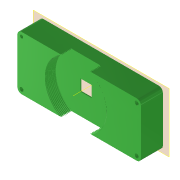
# Autodesk Inventor part: OutputFile
Saved by Autodesk Inventor 2022 (Build 260153000, 153)
## iProperties
Created: 2022-02-02
Part Number: OutputFile
Material: Generisch
Document SubType Name: Modeling
Designer: diederichbenedict
Density: 1 g/cm^3
Appearance: Glatt - Waldgrün
Mass: 24.3371 g
Surface Area: 140.293 cm^2
Volume: 24.3371 cm^3
Author: diederichbenedict
Autodesk Inventor part; units mm, degrees
ref_plane "YZ Plane" through (0, 0, 0) normal (1, 0, 0) x (0, 1, 0)
ref_plane "XZ Plane" through (0, 0, 0) normal (0, 1, 0) x (-1, 0, 0)
ref_plane "XY Plane" through (0, 0, 0) normal (0, 0, 1) x (1, 0, 0)
ref_plane "Arbeitsebene1" through (0, 0, 0) normal (0, 0, 1) x (1, 0, 0)
sketch "Skizze1" plane through (0, 0, 0) normal (0, 0, 1) x (1, 0, 0)
  line L0 (55.3299, 14.4874) -> (55.3299, -14.4874)
  line L1 (55.3299, -14.4874) -> (-23.745, -14.4874)
  line L2 (-23.745, -14.4874) -> (-23.745, 14.4874)
  line L3 (-23.745, 14.4874) -> (55.3299, 14.4874)
  line L4 (-3.798, -8.3739) -> (-3.798, -13.5126) projected
  line L5 (26.202, -8.3739) -> (-3.798, -8.3739) projected
  line L6 (-3.865, 8.7531) -> (26.135, 8.7531) projected
  line L7 (-3.865, 13.4874) -> (-3.865, 8.7531) projected
  line L8 (-3.865, 13.4874) -> (-14.255, 13.4874) projected
  arc A0 (-14.255, 13.4874) -> (-15.255, 12.4874) centre (-14.255, 12.4874) ccw projected
  line L9 (-15.255, 12.4874) -> (-15.255, -12.5126) projected
  arc A1 (-15.255, -12.5126) -> (-14.255, -13.5126) centre (-14.255, -12.5126) ccw projected
  line L10 (-14.255, -13.5126) -> (-3.798, -13.5126) projected
  arc A2 (-18.955, -12.5126) -> (-14.255, -17.2126) centre (-14.255, -12.5126) ccw projected
  line L11 (-18.955, -12.5126) -> (-18.955, 12.4874) projected
  arc A3 (-14.255, 17.1874) -> (-18.955, 12.4874) centre (-14.255, 12.4874) ccw projected
  line L12 (-14.255, 17.1874) -> (23.745, 17.1874) projected
  arc A4 (28.445, 12.4874) -> (23.745, 17.1874) centre (23.745, 12.4874) ccw projected
  arc A5 (23.745, -17.2126) -> (28.445, -12.5126) centre (23.745, -12.5126) ccw projected
  line L13 (23.745, -17.2126) -> (-14.255, -17.2126) projected
  circle A6 centre (57.3299, 16.4874) radius 1.4 projected
  circle A7 centre (-25.745, -16.4874) radius 1.4 projected
  circle A8 centre (57.3299, -16.4874) radius 1.4 projected
  circle A9 centre (-25.745, 16.4874) radius 1.15 projected
  line L14 (60.3299, 16.4874) -> (60.3299, -16.4874) projected
  arc A10 (60.3299, 16.4874) -> (57.3299, 19.4874) centre (57.3299, 16.4874) ccw projected
  line L15 (-25.745, 19.4874) -> (57.3299, 19.4874) projected
  arc A11 (-25.745, 19.4874) -> (-28.745, 16.4874) centre (-25.745, 16.4874) ccw projected
  line L16 (-28.745, -16.4874) -> (-28.745, 16.4874) projected
  arc A12 (-28.745, -16.4874) -> (-25.745, -19.4874) centre (-25.745, -16.4874) ccw projected
  line L17 (57.3299, -19.4874) -> (-25.745, -19.4874) projected
  arc A13 (57.3299, -19.4874) -> (60.3299, -16.4874) centre (57.3299, -16.4874) ccw projected
  arc A14 (-18.955, -12.5126) -> (-14.255, -17.2126) centre (-14.255, -12.5126) ccw projected
  line L18 (-18.955, -12.5126) -> (-18.955, 12.4874) projected
  arc A15 (-14.255, 17.1874) -> (-18.955, 12.4874) centre (-14.255, 12.4874) ccw projected
  line L19 (-14.255, 17.1874) -> (23.745, 17.1874) projected
  arc A16 (28.445, 12.4874) -> (23.745, 17.1874) centre (23.745, 12.4874) ccw projected
  line L20 (28.445, 12.4874) -> (26.135, 12.4874) projected
  line L21 (26.135, 8.7531) -> (26.135, 12.4874) projected
  line L22 (26.202, -12.5126) -> (26.202, -8.3739) projected
  line L23 (26.202, -12.5126) -> (28.445, -12.5126) projected
  arc A17 (23.745, -17.2126) -> (28.445, -12.5126) centre (23.745, -12.5126) ccw projected
  line L24 (23.745, -17.2126) -> (-14.255, -17.2126) projected
  circle A18 centre (57.3299, 16.4874) radius 1.4 projected
  circle A19 centre (-25.745, -16.4874) radius 1.4 projected
  circle A20 centre (57.3299, -16.4874) radius 1.4 projected
  circle A21 centre (-25.745, 16.4874) radius 1.15 projected
  line L25 (60.3299, 16.4874) -> (60.3299, -16.4874) projected
  arc A22 (60.3299, 16.4874) -> (57.3299, 19.4874) centre (57.3299, 16.4874) ccw projected
  line L26 (-25.745, 19.4874) -> (57.3299, 19.4874) projected
  arc A23 (-25.745, 19.4874) -> (-28.745, 16.4874) centre (-25.745, 16.4874) ccw projected
  line L27 (-28.745, -16.4874) -> (-28.745, 16.4874) projected
  arc A24 (-28.745, -16.4874) -> (-25.745, -19.4874) centre (-25.745, -16.4874) ccw projected
  line L28 (57.3299, -19.4874) -> (-25.745, -19.4874) projected
  arc A25 (57.3299, -19.4874) -> (60.3299, -16.4874) centre (57.3299, -16.4874) ccw projected
  line L29 (28.445, 12.4874) -> (26.135, 12.4874) projected
  line L30 (26.135, 8.7531) -> (26.135, 12.4874) projected
  line L31 (-3.865, 8.7531) -> (26.135, 8.7531) projected
  line L32 (-3.865, 13.4874) -> (-3.865, 8.7531) projected
  line L33 (-3.865, 13.4874) -> (-14.255, 13.4874) projected
  arc A26 (-14.255, 13.4874) -> (-15.255, 12.4874) centre (-14.255, 12.4874) ccw projected
  line L34 (-15.255, 12.4874) -> (-15.255, -12.5126) projected
  arc A27 (-15.255, -12.5126) -> (-14.255, -13.5126) centre (-14.255, -12.5126) ccw projected
  line L35 (-14.255, -13.5126) -> (-3.798, -13.5126) projected
  line L36 (-3.798, -8.3739) -> (-3.798, -13.5126) projected
  line L37 (26.202, -8.3739) -> (-3.798, -8.3739) projected
  line L38 (26.202, -12.5126) -> (26.202, -8.3739) projected
  line L39 (26.202, -12.5126) -> (28.445, -12.5126) projected
  point P0 (0, 0)
  point P1 (-15.255, 11.1874)
  point P2 (28.01, -14.4874)
  point P3 (-18.5199, -14.4874)
  point P4 (-18.5082, 14.4874)
  point P5 (27.9983, 14.4874)
  constraints: 8 end point
ref_plane "Arbeitsebene2" through (-3.9015, -6.25, 7.6898) normal (0, 0, 1) x (1, 0, 0)
extrude "Extrusion1" add sketch "Skizze1" along normal up to surface (7.6898 mm away)
sketch "Skizze2" plane through (-25.745, -19.4874, 7.6898) normal (0, 0, 1) x (1, 0, 0)
  line L0 (34.9935, 15.3874) -> (43.1935, 15.3874)
  line L1 (43.1935, 15.3874) -> (43.1935, 23.5874)
  line L2 (43.1935, 23.5874) -> (34.9935, 23.5874)
  line L3 (34.9935, 23.5874) -> (34.9935, 15.3874)
  line L4 (34.9935, 15.3874) -> (43.1935, 23.5874) construction
  line L5 (43.1935, 15.3874) -> (34.9935, 23.5874) construction
  line L6 (81.0749, 33.9749) -> (53.7433, 33.9749) projected
  line L7 (81.0749, 5) -> (81.0749, 33.9749) projected
  line L8 (53.755, 5) -> (81.0749, 5) projected
  arc A0 (49.4901, 2.2749) -> (53.755, 5) centre (49.4901, 6.9749) ccw projected
  line L9 (11.4901, 2.2749) -> (49.4901, 2.2749) projected
  arc A1 (7.2251, 5) -> (11.4901, 2.2749) centre (11.4901, 6.9749) ccw projected
  line L10 (2, 5) -> (7.2251, 5) projected
  line L11 (2, 33.9749) -> (2, 5) projected
  line L12 (7.2369, 33.9749) -> (2, 33.9749) projected
  arc A2 (11.4901, 36.6749) -> (7.2369, 33.9749) centre (11.4901, 31.9749) ccw projected
  line L13 (49.4901, 36.6749) -> (11.4901, 36.6749) projected
  arc A3 (53.7433, 33.9749) -> (49.4901, 36.6749) centre (49.4901, 31.9749) ccw projected
  circle A4 centre (83.0749, 35.9749) radius 1.4 projected
  circle A5 centre (0, 3) radius 1.4 projected
  circle A6 centre (83.0749, 3) radius 1.4 projected
  circle A7 centre (0, 35.9749) radius 1.15 projected
  arc A8 (0, 38.9749) -> (-3, 35.9749) centre (0, 35.9749) ccw projected
  line L14 (-3, 3) -> (-3, 35.9749) projected
  arc A9 (-3, 3) -> (0, 0) centre (0, 3) ccw projected
  line L15 (83.0749, 0) -> (0, 0) projected
  arc A10 (83.0749, 0) -> (86.0749, 3) centre (83.0749, 3) ccw projected
  line L16 (86.0749, 35.9749) -> (86.0749, 3) projected
  arc A11 (86.0749, 35.9749) -> (83.0749, 38.9749) centre (83.0749, 35.9749) ccw projected
  line L17 (0, 38.9749) -> (83.0749, 38.9749) projected
  circle A12 centre (39.0935, 19.4874) radius 3.6158 projected
  point P0 (25.745, 19.4874)
  dimension "d3" = 8.2
  dimension "d4" = 8.2
  constraints: 12 end point, 2 parallel, 1 horizontal, 1 perpendicular
  measures "d3" distance of L2.end L1.end
  measures "d4" distance of L1.end L0.end
extrude "Extrusion2" add sketch "Skizze2" along normal blind 2.2 contours L7 L8 A0 L9 A1 L10 L11 L12 A2 L13 A3 L6 | L17 A11 L16 A10 L15 A9 L14 A8
ref_plane "Arbeitsebene3" through (-21.9576, -12.7, 16.9028) normal (0, 0, -1) x (0, 1, 0)
sketch "Skizze3" plane through (-25.745, -19.4874, 9.8898) normal (0, 0, 1) x (1, 0, 0)
  line L0 (34.9935, 15.3874) -> (34.9935, 23.5874) projected
  line L1 (34.9935, 23.5874) -> (43.1935, 23.5874) projected
  line L2 (43.1935, 23.5874) -> (43.1935, 15.3874) projected
  line L3 (43.1935, 15.3874) -> (34.9935, 15.3874) projected
  circle A0 centre (39.0935, 19.4874) radius 3.6158 projected
  circle A1 centre (39.0935, 19.4874) radius 3.475
  line L4 (83.0749, 38.9749) -> (0, 38.9749) projected
  arc A2 (0, 38.9749) -> (-3, 35.9749) centre (0, 35.9749) ccw projected
  line L5 (-3, 35.9749) -> (-3, 3) projected
  arc A3 (-3, 3) -> (0, 0) centre (0, 3) ccw projected
  line L6 (0, 0) -> (83.0749, 0) projected
  arc A4 (83.0749, 0) -> (86.0749, 3) centre (83.0749, 3) ccw projected
  line L7 (86.0749, 3) -> (86.0749, 35.9749) projected
  arc A5 (86.0749, 35.9749) -> (83.0749, 38.9749) centre (83.0749, 35.9749) ccw projected
  line L8 (34.9935, 15.3874) -> (34.9935, 23.5874) projected
  line L9 (34.9935, 23.5874) -> (43.1935, 23.5874) projected
  line L10 (43.1935, 23.5874) -> (43.1935, 15.3874) projected
  line L11 (43.1935, 15.3874) -> (34.9935, 15.3874) projected
  circle A6 centre (0, 35.9749) radius 1.15 projected
  circle A7 centre (83.0749, 3) radius 1.4 projected
  circle A8 centre (0, 3) radius 1.4 projected
  circle A9 centre (83.0749, 35.9749) radius 1.4 projected
  point P0 (25.745, 19.4874)
  dimension "d7" = 6.95
  constraints: 1 centre point, 1 coincident
  measures "d7" diameter of A1
extrude "Extrusion3" add sketch "Skizze3" along normal blind 6 contours L0 L1 L2 L3 | A5 L7 A4 L6 A3 L5 A2 L4
sketch "Skizze4" plane through (-25.745, 19.4874, 15.8898) normal (0, 0, 1) x (1, 0, 0)
  circle A0 centre (39.0935, -19.4874) radius 3.6158 projected
  circle A1 centre (39.0935, -19.4874) radius 22
  point P0 (25.745, -19.4874)
  dimension "d10" = 44
  constraints: 1 centre point, 1 coincident
  measures "d10" diameter of A1
extrude "Extrusion4" cut sketch "Skizze4" against normal blind 7.5
sketch "Sketch7" plane through (13.3485, 22.5, 5.8898) normal (-1, 0, 0) x (0, 0, 1)
  line L0 (2.5, 0.2165) -> (2.3389, -0.0625) construction
  line L1 (2.5, 0.2165) -> (2.6611, -0.0625) construction
  line L2 (2.5, 0.2165) -> (2.5, 0) construction
  line L3 (2.375, 0) -> (2.4472, 0) construction
  line L4 (3, -0.6495) -> (3.0625, -0.5413) construction
  line L5 (2, -0.6495) -> (1.9375, -0.5413) construction
  line L6 (1.9375, -0.5413) -> (2, -0.5413) construction
  line L7 (2.0625, -0.5413) -> (2, -0.6495) construction
  arc A0 (2.4472, 0) -> (2.3389, -0.0625) centre (2.4472, -0.125) ccw
  arc A1 (2.6611, -0.0625) -> (2.5528, 0) centre (2.5528, -0.125) ccw
  line L8 (3, -0.6495) -> (3, -0.5413) construction
  line L9 (2, -0.6495) -> (2, -0.5413) construction
  arc A2 (2.9195, -0.51) -> (2.9736, -0.5413) centre (2.9736, -0.4788) ccw
  line L10 (2.6611, -0.0625) -> (2.9195, -0.51)
  line L11 (2.4472, 0) -> (2.5528, 0)
  line L12 (2.3389, -0.0625) -> (2.0805, -0.51)
  line L13 (2.9736, -0.5413) -> (3, -0.5413) construction
  line L14 (3, -0.5413) -> (3.0625, -0.5413) construction
  arc A3 (2.0264, -0.5413) -> (2.0805, -0.51) centre (2.0264, -0.4788) ccw
  line L15 (2.0805, -0.51) -> (2.0625, -0.5413) construction
  line L16 (2, -0.5413) -> (2.0264, -0.5413) construction
  line L17 (2.0264, -0.5413) -> (2.9736, -0.5413)
  line L18 (0, 0) -> (0.4413, 0)
  line L19 (0, 0) -> (0, 0.419)
  line L20 (3, -0.6495) -> (2.9195, -0.51) construction
  dimension "d41" = 0.2165
  dimension "d42" = 0.125
  dimension "d43" = 0.0625
  dimension "d44" = 0.1082
  dimension "d45" = 1
  dimension "Sketch7_MajorRadius" = 0.5413
  dimension "d47" = 60
  dimension "Sketch7_ThreadOffset" = 3
  dimension "Sketch7_MinorRadius" = 0
  constraints: 42 end point, 17 tangent, 8 point on circle, 6 parallel, 5 collinear, 4 centre point, 3 point on line, 2 equal radius, 2 horizontal, 2 perpendicular, 2 vertical, 1 equal length, 1 midpoint, 4 other
  measures "d41" distance from line of L0.start L3
  measures "d42" radius of A0
  measures "d43" radius of A2
  measures "d44" distance from line of L14 L4.start
  measures "d45" distance between parallel lines of L8 L9
  measures "Sketch7_MajorRadius" distance between parallel lines of L14 L18
  measures "d47" angle of L10 L12
  measures "Sketch7_ThreadOffset" distance between parallel lines of L19 L8
  measures "Sketch7_MinorRadius" distance between parallel lines of L18 L11
thread "Gewinde1" size "M45x1" class "6H" standard "ANSI Metric M Profile" full length
sketch "Skizze10" plane through (-25.745, -19.4874, 7.6898) normal (0, 0, -1) x (-1, 0, 0)
  arc A0 (-50.4901, 6.9749) -> (-49.4901, 5.9749) centre (-49.4901, 6.9749) ccw projected
  line L0 (-49.4901, 5.9749) -> (-11.4901, 5.9749) projected
  arc A1 (-11.4901, 5.9749) -> (-10.4901, 6.9749) centre (-11.4901, 6.9749) ccw projected
  line L1 (-10.4901, 6.9749) -> (-10.4901, 31.9749) projected
  arc A2 (-10.4901, 31.9749) -> (-11.4901, 32.9749) centre (-11.4901, 31.9749) ccw projected
  line L2 (-11.4901, 32.9749) -> (-49.4901, 32.9749) projected
  arc A3 (-49.4901, 32.9749) -> (-50.4901, 31.9749) centre (-49.4901, 31.9749) ccw projected
  line L3 (-50.4901, 31.9749) -> (-50.4901, 6.9749) projected
  line L4 (3, 35.9749) -> (3, 3) projected
  arc A4 (3, 35.9749) -> (0, 38.9749) centre (0, 35.9749) ccw projected
  line L5 (-83.0749, 38.9749) -> (0, 38.9749) projected
  arc A5 (-83.0749, 38.9749) -> (-86.0749, 35.9749) centre (-83.0749, 35.9749) ccw projected
  line L6 (-86.0749, 3) -> (-86.0749, 35.9749) projected
  arc A6 (-86.0749, 3) -> (-83.0749, 0) centre (-83.0749, 3) ccw projected
  line L7 (0, 0) -> (-83.0749, 0) projected
  arc A7 (0, 0) -> (3, 3) centre (0, 3) ccw projected
  circle A8 centre (0, 35.9749) radius 1.15 projected
  circle A9 centre (-83.0749, 3) radius 1.4 projected
  circle A10 centre (0, 3) radius 1.4 projected
  circle A11 centre (-83.0749, 35.9749) radius 1.4 projected
  line L8 (-81.0749, 33.9749) -> (-81.0749, 5) projected
  line L9 (-53.7433, 33.9749) -> (-81.0749, 33.9749) projected
  arc A12 (-49.4901, 36.6749) -> (-53.7433, 33.9749) centre (-49.4901, 31.9749) ccw projected
  line L10 (-11.4901, 36.6749) -> (-49.4901, 36.6749) projected
  arc A13 (-7.2369, 33.9749) -> (-11.4901, 36.6749) centre (-11.4901, 31.9749) ccw projected
  line L11 (-2, 33.9749) -> (-7.2369, 33.9749) projected
  line L12 (-2, 5) -> (-2, 33.9749) projected
  line L13 (-7.2251, 5) -> (-2, 5) projected
  arc A14 (-11.4901, 2.2749) -> (-7.2251, 5) centre (-11.4901, 6.9749) ccw projected
  line L14 (-49.4901, 2.2749) -> (-11.4901, 2.2749) projected
  arc A15 (-53.755, 5) -> (-49.4901, 2.2749) centre (-49.4901, 6.9749) ccw projected
  line L15 (-81.0749, 5) -> (-53.755, 5) projected
  line L16 (-6.7901, 31.9749) -> (-6.7901, 6.9749)
  arc A16 (-11.4901, 2.2749) -> (-6.7901, 6.9749) centre (-11.4901, 6.9749) ccw
  line L17 (-11.4901, 2.2749) -> (-49.4901, 2.2749)
  arc A17 (-54.1901, 6.9749) -> (-49.4901, 2.2749) centre (-49.4901, 6.9749) ccw
  line L18 (-54.1901, 6.9749) -> (-54.1901, 31.9749)
  arc A18 (-49.4901, 36.6749) -> (-54.1901, 31.9749) centre (-49.4901, 31.9749) ccw
  line L19 (-49.4901, 36.6749) -> (-11.4901, 36.6749)
  arc A19 (-6.7901, 31.9749) -> (-11.4901, 36.6749) centre (-11.4901, 31.9749) ccw
  line L20 (-10.6401, 31.9749) -> (-10.6401, 6.9749)
  arc A20 (-11.4901, 6.1249) -> (-10.6401, 6.9749) centre (-11.4901, 6.9749) ccw
  line L21 (-11.4901, 6.1249) -> (-49.4901, 6.1249)
  arc A21 (-50.3401, 6.9749) -> (-49.4901, 6.1249) centre (-49.4901, 6.9749) ccw
  line L22 (-50.3401, 6.9749) -> (-50.3401, 31.9749)
  arc A22 (-49.4901, 32.8249) -> (-50.3401, 31.9749) centre (-49.4901, 31.9749) ccw
  line L23 (-49.4901, 32.8249) -> (-11.4901, 32.8249)
  arc A23 (-10.6401, 31.9749) -> (-11.4901, 32.8249) centre (-11.4901, 31.9749) ccw
  point P0 (-25.745, 19.4874)
  point P1 (-53.755, 5)
  dimension "d72" = 0.15
  constraints: 17 point on circle, 16 end point, 8 centre point, 14 other
  measures "d72" distance between parallel lines of L1 L20
extrude "Extrusion6" add sketch "Skizze10" along normal blind 3 contours L3 A3 L2 A2 L1 A1 L0 A0 | A12 L10 A13 A19 L16 A16 A14 L14 A15 A17 L18 A18
coil "Spirale4" sketch "Sketch7" operation cut axis through (13.3485, 0, 15.8898) along (0, 0, 1) pitch 1.001 turns 9.99001 hand right
sketch "Skizze11" plane through (-25.745, -19.4874, 4.6898) normal (0, 0, -1) x (-1, 0, 0)
  arc A0 (-6.7901, 31.9749) -> (-7.2369, 33.9749) centre (-11.4901, 31.9749) ccw projected
  arc A1 (-7.2369, 33.9749) -> (-11.4901, 36.6749) centre (-11.4901, 31.9749) ccw projected
  line L0 (-49.4901, 36.6749) -> (-11.4901, 36.6749) projected
  arc A2 (-49.4901, 36.6749) -> (-53.7433, 33.9749) centre (-49.4901, 31.9749) ccw projected
  arc A3 (-53.7433, 33.9749) -> (-54.1901, 31.9749) centre (-49.4901, 31.9749) ccw projected
  line L1 (-54.1901, 31.9749) -> (-54.1901, 6.9749) projected
  arc A4 (-54.1901, 6.9749) -> (-53.755, 5) centre (-49.4901, 6.9749) ccw projected
  arc A5 (-53.755, 5) -> (-49.4901, 2.2749) centre (-49.4901, 6.9749) ccw projected
  line L2 (-11.4901, 2.2749) -> (-49.4901, 2.2749) projected
  arc A6 (-11.4901, 2.2749) -> (-7.2251, 5) centre (-11.4901, 6.9749) ccw projected
  arc A7 (-7.2251, 5) -> (-6.7901, 6.9749) centre (-11.4901, 6.9749) ccw projected
  line L3 (-6.7901, 6.9749) -> (-6.7901, 31.9749) projected
  line L4 (-49.4901, 32.8249) -> (-11.4901, 32.8249) projected
  arc A8 (-10.6401, 31.9749) -> (-11.4901, 32.8249) centre (-11.4901, 31.9749) ccw projected
  line L5 (-10.6401, 31.9749) -> (-10.6401, 6.9749) projected
  arc A9 (-11.4901, 6.1249) -> (-10.6401, 6.9749) centre (-11.4901, 6.9749) ccw projected
  line L6 (-11.4901, 6.1249) -> (-49.4901, 6.1249) projected
  arc A10 (-50.3401, 6.9749) -> (-49.4901, 6.1249) centre (-49.4901, 6.9749) ccw projected
  line L7 (-50.3401, 6.9749) -> (-50.3401, 31.9749) projected
  arc A11 (-49.4901, 32.8249) -> (-50.3401, 31.9749) centre (-49.4901, 31.9749) ccw projected
  line L8 (-54.1901, 31.9749) -> (-54.1901, 6.9749) projected
  line L9 (-54.1901, 31.9749) -> (-50.3401, 31.9749)
  line L10 (-50.3401, 31.9749) -> (-50.3401, 6.9749)
  line L11 (-50.3401, 6.9749) -> (-54.1901, 6.9749)
  line L12 (-54.1901, 6.9749) -> (-54.1901, 31.9749)
  point P0 (-25.745, 19.4874)
  point P1 (-54.1901, 6.9749)
  constraints: 8 end point, 2 parallel, 1 horizontal, 1 perpendicular
extrude "Extrusion7" cut sketch "Skizze11" against normal up to surface (3 mm away) contours L9 L7 L11 L1
equation "\"d41\" = 0.216506 * Sketch7_Pitch"
equation "\"d42\" = d50"
equation "\"d43\" = 0.0625 * Sketch7_Pitch"
equation "\"d44\" = 0.108253 * Sketch7_Pitch"
equation "\"d45\" = Sketch7_Pitch"
equation "\"d47\" = d52"
equation "\"d50\" = 0.125 * Sketch7_Pitch"
equation "\"Sketch7_Pitch\" = 1"
equation "\"d52\" = 60deg"
